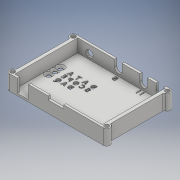
# Autodesk Inventor part: Redid Enclosure Top
Saved by Autodesk Inventor 2017 (Build 210142000, 142)
## iProperties
Created: 2017-07-24
Part Number: Redid Enclosure Top
Material: Generic
Document SubType Name: Modeling
Designer: andrew
Density: 1 g/cm^3
Appearance: Default
Author: andrew
Autodesk Inventor part; units mm, degrees
ref_plane "YZ Plane" through (0, 0, 0) normal (1, 0, 0) x (0, 1, 0)
ref_plane "XZ Plane" through (0, 0, 0) normal (0, 1, 0) x (-1, 0, 0)
ref_plane "XY Plane" through (0, 0, 0) normal (0, 0, 1) x (1, 0, 0)
sketch "Sketch1" plane through (0, 0, 0) normal (0, 0, 1) x (1, 0, 0)
  line L0 (85.72, 30.226) -> (85.72, 1.401) construction
  line L1 (85.72, 1.401) -> (45.72, 1.401) construction
  line L2 (85.72, 1.401) -> (5.72, 1.401) construction
  line L3 (5.72, 1.401) -> (5.72, 59.001) construction
  line L4 (5.72, 59.001) -> (85.72, 59.001) construction
  line L5 (85.72, 59.001) -> (85.72, 1.401) construction
  line L6 (61.99, 1.401) -> (61.99, 20.221) construction
  line L7 (61.99, 20.221) -> (85.72, 20.221) construction
  line L8 (61.99, 20.221) -> (58.44, 20.221) construction
  line L9 (61.99, 23.771) -> (61.99, 20.221) construction
  line L10 (60.215, 20.221) -> (61.99, 20.221) construction
  line L11 (61.99, 20.221) -> (61.99, 21.996) construction
  line L12 (61.99, 21.996) -> (60.215, 21.996) construction
  line L13 (60.215, 21.996) -> (60.215, 20.221) construction
  circle A0 centre (60.215, 21.996) radius 1.775 construction
  circle A1 centre (60.215, 21.996) radius 2.775 construction
  circle A2 centre (60.215, 21.996) radius 4.275 construction
  line L14 (5.72, 59.001) -> (74.72, 59.001) construction
  line L15 (74.72, 59.001) -> (74.72, 53.301) construction
  line L16 (74.72, 53.301) -> (5.72, 53.301) construction
  line L17 (5.72, 53.301) -> (5.72, 59.001) construction
  line L18 (5.72, 1.401) -> (18.72, 1.401) construction
  line L19 (18.72, 1.401) -> (18.72, 14.401) construction
  line L20 (18.72, 14.401) -> (5.72, 14.401) construction
  line L21 (5.72, 14.401) -> (5.72, 1.401) construction
  circle A3 centre (2.72, 58.001) radius 2
  line L22 (3.72, 61.001) -> (5.72, 61.001)
  line L23 (5.72, 61.001) -> (5.72, 59.001) construction
  line L24 (5.72, 61.001) -> (2.72, 61.001)
  line L25 (5.72, 55.001) -> (5.72, 61.001) construction
  line L26 (45.72, 1.9437) -> (45.72, 30.226) construction
  line L27 (45.72, 30.226) -> (85.72, 30.226) construction
  arc A4 (2.72, 61.001) -> (1.52, 55.2515) centre (2.72, 58.001) ccw
  circle A5 centre (2.72, 2.451) radius 2
  line L28 (3.72, -0.549) -> (5.72, -0.549)
  line L29 (5.72, -0.549) -> (2.72, -0.549)
  arc A6 (1.52, 5.2005) -> (2.72, -0.549) centre (2.72, 2.451) ccw
  circle A7 centre (88.72, 58.001) radius 2
  line L30 (85.72, 61.001) -> (88.72, 61.001)
  arc A8 (89.92, 55.2515) -> (88.72, 61.001) centre (88.72, 58.001) ccw
  line L31 (85.72, -0.549) -> (88.72, -0.549)
  circle A9 centre (88.72, 2.451) radius 2
  arc A10 (88.72, -0.549) -> (89.92, 5.2005) centre (88.72, 2.451) ccw
  line L32 (2.72, 53.4184) -> (2.72, 7.0336)
  line L33 (5.72, 61.001) -> (85.72, 61.001)
  line L34 (88.72, 53.4184) -> (88.72, 7.0336)
  line L35 (85.72, -0.549) -> (5.72, -0.549)
  arc A11 (2.72, 53.4184) -> (1.52, 55.2515) centre (0.72, 53.4184) ccw
  arc A12 (1.52, 5.2005) -> (2.72, 7.0336) centre (0.72, 7.0336) ccw
  arc A13 (88.72, 7.0336) -> (89.92, 5.2005) centre (90.72, 7.0336) ccw
  arc A14 (89.92, 55.2515) -> (88.72, 53.4184) centre (90.72, 53.4184) ccw
  point P0 (0, 0)
  point P1 (2.72, 55.001)
  point P2 (2.72, 5.451)
  point P3 (91.44, 0)
  point P4 (88.72, 55.001)
  point P5 (88.72, 5.451)
  dimension "d32" = 40
  dimension "d33" = 28.825
  dimension "d34" = 80
  dimension "d37" = 18.82
  dimension "d40" = 5.55
  dimension "d41" = 8.55
  dimension "d42" = 69
  dimension "d43" = 5.7
  dimension "d44" = 13
  dimension "d45" = 13
  dimension "d52" = 2
  dimension "d80" = 4
  constraints: 72 end point, 20 point on circle, 17 symmetric about line, 14 centre point, 9 parallel, 8 tangent, 7 perpendicular, 6 horizontal, 6 point on line, 3 coincident, 3 equal radius, 2 midpoint, 2 vertical, 1 horizontal alignment, 8 other
  measures "d32" distance of L0.end L1.end
  measures "d33" distance of L0.start L0.end
  measures "d34" distance of L3.end L4.end
  measures "d37" distance of L6.start L6.end
  measures "d40" diameter of A1
  measures "d41" diameter of A2
  measures "d42" distance of L15.end L16.end
  measures "d43" distance of L14.end L15.end
  measures "d44" distance of L20.end L19.end
  measures "d45" distance of L19.end L18.end
  measures "d52" radius of A11
  measures "d80" diameter of A3
extrude "Extrusion1" add sketch "Sketch1" along normal blind 2
sketch "Sketch2" plane through (0, 0, 2) normal (0, 0, 1) x (1, 0, 0)
  line L0 (85.72, 30.226) -> (85.72, 1.401)
  line L1 (5.72, 14.401) -> (5.72, 53.301)
  line L2 (74.72, 59.001) -> (85.72, 59.001)
  line L3 (85.72, 59.001) -> (85.72, 1.401)
  line L4 (45.72, 59.001) -> (74.72, 59.001)
  line L5 (5.72, 58.001) -> (5.72, 59.001)
  line L6 (5.72, 1.401) -> (18.72, 1.401)
  line L7 (5.72, 2.451) -> (5.72, 1.401)
  circle A0 centre (2.72, 58.001) radius 2
  line L8 (3.72, 61.001) -> (5.72, 61.001)
  line L9 (5.72, 61.001) -> (5.72, 59.001)
  line L10 (5.72, 61.001) -> (2.72, 61.001)
  line L11 (5.72, 59.001) -> (5.72, 61.001)
  arc A1 (2.72, 61.001) -> (1.52, 55.2515) centre (2.72, 58.001) ccw
  line L12 (3.72, -0.549) -> (5.72, -0.549)
  line L13 (5.72, -0.549) -> (2.72, -0.549)
  circle A2 centre (2.72, 2.451) radius 2
  arc A3 (1.52, 5.2005) -> (2.72, -0.549) centre (2.72, 2.451) ccw
  line L14 (85.72, -0.549) -> (88.72, -0.549)
  circle A4 centre (88.72, 2.451) radius 2
  arc A5 (88.72, -0.549) -> (89.92, 5.2005) centre (88.72, 2.451) ccw
  circle A6 centre (88.72, 58.001) radius 2
  arc A7 (89.92, 55.2515) -> (88.72, 61.001) centre (88.72, 58.001) ccw
  line L15 (85.72, 61.001) -> (88.72, 61.001)
  line L16 (2.72, 53.4184) -> (2.72, 7.0336)
  line L17 (5.72, 61.001) -> (85.72, 61.001)
  line L18 (88.72, 53.4184) -> (88.72, 7.0336)
  line L19 (85.72, -0.549) -> (5.72, -0.549)
  arc A8 (2.72, 53.4184) -> (1.52, 55.2515) centre (0.72, 53.4184) ccw
  arc A9 (1.52, 5.2005) -> (2.72, 7.0336) centre (0.72, 7.0336) ccw
  arc A10 (88.72, 7.0336) -> (89.92, 5.2005) centre (90.72, 7.0336) ccw
  arc A11 (89.92, 55.2515) -> (88.72, 53.4184) centre (90.72, 53.4184) ccw
  line L20 (85.72, 1.401) -> (74.72, 1.401)
  line L21 (61.99, 1.401) -> (45.72, 1.401)
  line L22 (85.72, 1.401) -> (74.72, 1.401)
  line L23 (61.99, 1.401) -> (18.72, 1.401)
  line L24 (61.99, 1.401) -> (74.72, 1.401)
  line L25 (5.72, 14.401) -> (5.72, 2.451)
  line L26 (5.72, 53.301) -> (5.72, 58.001)
  line L27 (5.72, 59.001) -> (45.72, 59.001)
  point P0 (0, 0)
  point P1 (2.72, 55.001)
  point P2 (2.72, 5.451)
  point P3 (91.44, 0)
  point P4 (88.72, 5.451)
  point P5 (88.72, 55.001)
  dimension "d53" = 40
  dimension "d54" = 28.825
  dimension "d55" = 80
  dimension "d63" = 2
  dimension "d81" = 4
  dimension "d82" = 4
  dimension "d83" = 4
  dimension "d84" = 4
  constraints: 56 end point, 22 point on circle, 12 centre point, 8 tangent, 6 horizontal, 4 parallel, 4 point on line, 3 equal radius, 3 perpendicular, 2 collinear, 2 vertical
  measures "d53" distance of L0.end L21.end
  measures "d54" distance of L0.start L0.end
  measures "d55" distance of L5.end L3.start
  measures "d63" radius of A8
  measures "d81" diameter of A0
  measures "d82" diameter of A2
  measures "d83" diameter of A4
  measures "d84" diameter of A6
extrude "Extrusion2" add sketch "Sketch2" along normal blind 12
sketch "Sketch6" plane through (2.72, 61.001, 0) normal (0, 1, 0) x (1, 0, 0)
  line L0 (36.777, -7.7431) -> (36.777, -7.7246)
  line L1 (43.7769, -7.7246) -> (43.7769, -7.7431)
  arc A0 (43.7769, -7.7431) -> (36.777, -7.7431) centre (40.2769, -7.7227) ccw
  arc A1 (66.82, -7.7246) -> (59.82, -7.7246) centre (63.32, -7.7246) ccw
  arc A2 (81.679, -7.7246) -> (74.679, -7.7246) centre (78.179, -7.7246) ccw
  line L2 (88.72, -8.9422) -> (88.72, 1.0414) construction
  line L3 (-2.72, 0.0414) -> (-2.72, -13.4714) construction
  arc A3 (11.6348, -3.8321) -> (15.9452, -3.8321) centre (13.79, -6.4991) ccw
  line L4 (11.6347, -3.8321) -> (15.9453, -3.8321)
  line L5 (-3, 0) -> (-3, -14) construction
  line L6 (89, 0) -> (89, -14) construction
  line L7 (-3, -7.115) -> (89, -7.115) construction
  line L8 (43, -7.115) -> (43, 6.037) construction
  line L9 (-2.72, -7.115) -> (43, -7.115) construction
  line L10 (47.3567, 23.0307) -> (47.3567, 24.0307)
  line L11 (43, -7.7246) -> (43.7769, -7.7246)
  line L12 (43.7769, -7.7246) -> (43.7769, -19.8521)
  line L13 (43.7769, -19.8521) -> (36.777, -19.8521)
  line L14 (36.777, -19.8521) -> (36.777, -7.7246)
  line L15 (66.82, -7.7246) -> (66.82, -18.3429)
  line L16 (66.82, -18.3429) -> (59.82, -18.3429)
  line L17 (59.82, -18.3429) -> (59.82, -7.7246)
  line L18 (81.679, -7.7246) -> (81.679, -19.1335)
  line L19 (81.679, -19.1335) -> (74.679, -19.1335)
  line L20 (74.679, -19.1335) -> (74.679, -7.7246)
  line L21 (96.4599, -13.1902) -> (96.4599, -14.5902)
  point P0 (-2.72, 0)
  dimension "d91" = 1
  dimension "d92" = 7
  dimension "d93" = 7
  dimension "d94" = 7
  dimension "d141" = 1.4
  constraints: 42 end point, 9 point on circle, 8 point on line, 4 centre point, 4 parallel, 3 vertical, 1 horizontal, 1 midpoint, 1 perpendicular
  measures "d91" distance of L10.start L10.end
  measures "d92" diameter of A0
  measures "d93" diameter of A1
  measures "d94" diameter of A2
  measures "d141" distance of L21.start L21.end
extrude "Extrusion6" cut sketch "Sketch6" against normal blind 10
sketch "Sketch7" plane through (2.72, -0.549, 0) normal (0, -1, 0) x (1, 0, 0)
  line L0 (36.015, 10.636) -> (36.015, 12.9729) construction
  line L1 (7.948, 2) -> (7.948, 12.9729) construction
  line L2 (-2.72, -0.54) -> (-2.72, 13.43) construction
  line L3 (88.72, -0.54) -> (88.72, 12.0462) construction
  line L4 (-2.72, 13.43) -> (88.72, 13.43) construction
  line L5 (43, 13.43) -> (43, 23.4779) construction
  line L6 (0, 14) -> (86, 14) construction
  line L7 (83, 14) -> (3, 14) construction
  line L8 (43, 14) -> (43, 26.0617) construction
  line L9 (36.015, 10.636) -> (36.015, 15.6286)
  line L10 (36.015, 15.6286) -> (49.35, 15.6286)
  line L11 (7.948, 2) -> (7.948, 16.2504)
  line L12 (7.948, 16.2504) -> (17.092, 16.2504)
  line L13 (35.515, 10.8) -> (49.85, 10.8)
  line L14 (49.85, 10.8) -> (49.85, 16.1286)
  line L15 (49.85, 16.1286) -> (35.515, 16.1286)
  line L16 (35.515, 16.1286) -> (35.515, 10.8)
  line L17 (7.448, 2) -> (17.592, 2)
  line L18 (17.592, 2) -> (17.592, 16.7504)
  line L19 (17.592, 16.7504) -> (7.448, 16.7504)
  line L20 (7.448, 16.7504) -> (7.448, 2)
  point P0 (-2.72, 0)
  point P1 (43, 12.16)
  dimension "d101" = 3.2
  dimension "d102" = 12
  constraints: 38 end point, 4 parallel, 2 midpoint, 2 perpendicular, 2 vertical, 1 horizontal, 2 other
  measures "d101" distance between parallel lines of L13 L6
  measures "d102" distance between parallel lines of L6 L17
extrude "Extrusion7" cut sketch "Sketch7" against normal blind 10
sketch "Sketch8" plane through (0, 0, 0) normal (0, 0, -1) x (-1, 0, 0)
  arc A0 (-89.92, 5.2005) -> (-88.72, -0.549) centre (-88.72, 2.451) ccw construction
  line L0 (-91.6567, 1.8381) -> (-82.1567, 1.8381) construction
  line L1 (-20.312, 1.401) -> (-85.72, 1.401) construction
  line L2 (-91.6567, 1.8381) -> (-82.1567, 1.8381) construction
  line L3 (-82.1567, -0.549) -> (-82.1567, 5.751) construction
  line L4 (-82.1567, 5.751) -> (-78.6567, 5.751) construction
  line L5 (-78.6567, 5.751) -> (-78.6567, 9.251) construction
  line L6 (-78.6567, 9.251) -> (-82.1567, 9.251) construction
  line L7 (-82.1567, 9.251) -> (-82.1567, 5.751) construction
  circle A1 centre (-80.4067, 7.501) radius 1.75
  line L8 (-84.399, 59.001) -> (-77.399, 59.001) construction
  line L9 (-84.399, 61.001) -> (-84.399, 59.001) construction
  line L10 (-77.399, 61.001) -> (-84.399, 61.001) construction
  line L11 (-77.399, 61.001) -> (-77.399, 59.001) construction
  line L12 (-69.54, 59.001) -> (-62.54, 59.001) construction
  line L13 (-69.54, 61.001) -> (-69.54, 59.001) construction
  line L14 (-62.54, 61.001) -> (-69.54, 61.001) construction
  line L15 (-62.54, 61.001) -> (-62.54, 59.001) construction
  line L16 (-46.4969, 59.001) -> (-39.497, 59.001) construction
  line L17 (-46.4969, 61.001) -> (-46.4969, 59.001) construction
  line L18 (-39.497, 61.001) -> (-46.4969, 61.001) construction
  line L19 (-39.497, 61.001) -> (-39.497, 59.001) construction
  line L20 (-88.72, 61.001) -> (-2.72, 61.001) construction
  line L21 (-80.899, 61.001) -> (-80.899, 58.001) construction
  line L22 (-80.899, 61.001) -> (-77.899, 61.001) construction
  line L23 (-66.04, 61.001) -> (-66.04, 58.001) construction
  line L24 (-42.9969, 61.001) -> (-42.9969, 58.001) construction
  line L25 (-81.6541, 57.9429) -> (-78.5881, 57.9429) construction
  line L26 (-78.5881, 57.9429) -> (-78.5881, 54.4344) construction
  line L27 (-78.5881, 54.4344) -> (-81.6541, 54.4344) construction
  line L28 (-81.6541, 54.4344) -> (-81.6541, 57.9429) construction
  line L29 (-44.9835, 57.8582) -> (-36.2955, 57.8582) construction
  line L30 (-36.2955, 57.8582) -> (-36.2955, 54.005) construction
  line L31 (-36.2955, 54.005) -> (-44.9835, 54.005) construction
  line L32 (-44.9835, 54.005) -> (-44.9835, 57.8582) construction
  line L33 (-68.3878, 54.2701) -> (-68.3878, 58.1234) construction
  line L34 (-68.3878, 58.1234) -> (-59.6998, 58.1234) construction
  line L35 (-59.6998, 58.1234) -> (-59.6998, 54.2701) construction
  line L36 (-59.6998, 54.2701) -> (-68.3878, 54.2701) construction
  arc A2 (-1.52, 55.2515) -> (-2.72, 61.001) centre (-2.72, 58.001) ccw construction
  line L37 (0.28, 58.001) -> (-7.5071, 58.001) construction
  line L38 (-85.72, 59.001) -> (-5.72, 59.001) construction
  line L39 (0.28, 58.001) -> (8.0671, 58.001) construction
  line L40 (-7.5071, 61.001) -> (-7.5071, 41.501) construction
  line L41 (-7.5071, 41.501) -> (-11.0671, 41.501) construction
  line L42 (-11.0671, 41.501) -> (-11.0671, 37.941) construction
  line L43 (-11.0671, 37.941) -> (-7.5071, 37.941) construction
  line L44 (-7.5071, 37.941) -> (-7.5071, 41.501) construction
  line L45 (-7.5071, 61.001) -> (-7.5071, 36.381) construction
  line L46 (-7.5071, 61.001) -> (17.1129, 61.001) construction
  line L47 (-7.5071, 36.381) -> (-11.0671, 36.381) construction
  line L48 (-11.0671, 36.381) -> (-11.0671, 32.821) construction
  line L49 (-11.0671, 32.821) -> (-7.5071, 32.821) construction
  line L50 (-7.5071, 32.821) -> (-7.5071, 36.381) construction
  line L51 (-7.5071, 61.001) -> (-7.5071, 30.621) construction
  line L52 (-7.5071, 30.621) -> (-11.0671, 30.621) construction
  line L53 (-11.0671, 30.621) -> (-11.0671, 27.061) construction
  line L54 (-11.0671, 27.061) -> (-7.5071, 27.061) construction
  line L55 (-7.5071, 27.061) -> (-7.5071, 30.621) construction
  circle A3 centre (-9.2871, 39.721) radius 1.78
  circle A4 centre (-9.2871, 34.601) radius 1.78
  circle A5 centre (-9.2871, 28.841) radius 1.78
  line L56 (-42.0074, 37.4126) -> (-42.0074, 41.2658) construction
  line L57 (-42.0074, 41.2658) -> (-11.5337, 41.2658) construction
  line L58 (-11.5337, 41.2658) -> (-11.5337, 37.4126) construction
  line L59 (-11.5337, 37.4126) -> (-42.0074, 37.4126) construction
  line L60 (-41.4894, 32.436) -> (-41.4894, 36.2892) construction
  line L61 (-41.4894, 36.2892) -> (-11.0157, 36.2892) construction
  line L62 (-11.0157, 36.2892) -> (-11.0157, 32.436) construction
  line L63 (-11.0157, 32.436) -> (-41.4894, 32.436) construction
  line L64 (-31.8137, 26.6882) -> (-31.8137, 30.5415) construction
  line L65 (-31.8137, 30.5415) -> (-1.34, 30.5415) construction
  line L66 (-1.34, 30.5415) -> (-1.34, 26.6882) construction
  line L67 (-1.34, 26.6882) -> (-31.8137, 26.6882) construction
  line L68 (-80.3543, 53.7647) -> (-81.2943, 53.7647)
  line L69 (-81.2943, 53.7647) -> (-81.2943, 57.9429)
  line L70 (-81.2943, 57.9429) -> (-80.3543, 57.9429)
  line L71 (-80.3543, 57.9429) -> (-80.3543, 53.7647)
  line L72 (-67.088, 53.9451) -> (-68.028, 53.9451)
  line L73 (-68.028, 53.9451) -> (-68.028, 58.1234)
  line L74 (-68.028, 58.1234) -> (-67.088, 58.1234)
  line L75 (-67.088, 58.1234) -> (-67.088, 53.9451)
  line L76 (-63.8173, 53.9451) -> (-64.7574, 53.9451)
  line L77 (-64.7574, 53.9451) -> (-64.7574, 58.1234)
  line L78 (-64.7574, 58.1234) -> (-63.8173, 58.1234)
  line L79 (-63.8173, 58.1234) -> (-63.8173, 53.9451)
  spline S0 degree 2 poles (-43.3336, 53.7156) (-43.7939, 53.7156) (-44.4876, 53.8939) (-44.7858, 54.0235) knots 0 0 0 1 2 2 2
  line L80 (-44.7858, 54.0235) -> (-44.7858, 54.9765)
  line L81 (-44.7858, 54.9765) -> (-44.695, 54.9765)
  spline S1 degree 2 poles (-44.695, 54.9765) (-44.3936, 54.7205) (-43.6707, 54.4449) (-43.3304, 54.4449) knots 0 0 0 1 2 2 2
  spline S2 degree 2 poles (-43.3304, 54.4449) (-43.2428, 54.4449) (-42.9608, 54.4838) (-42.8765, 54.5227) knots 0 0 0 1 2 2 2
  spline S3 degree 2 poles (-42.8765, 54.5227) (-42.7728, 54.5681) (-42.627, 54.7334) (-42.627, 54.8663) knots 0 0 0 1 2 2 2
  spline S4 degree 2 poles (-42.627, 54.8663) (-42.627, 55.0187) (-42.8636, 55.2067) (-43.0257, 55.2488) knots 0 0 0 1 2 2 2
  spline S5 degree 2 poles (-43.0257, 55.2488) (-43.2299, 55.3039) (-43.6934, 55.3979) (-43.8976, 55.4693) knots 0 0 0 1 2 2 2
  spline S6 degree 2 poles (-43.8976, 55.4693) (-44.3612, 55.6313) (-44.7631, 56.1856) (-44.7631, 56.6005) knots 0 0 0 1 2 2 2
  spline S7 degree 2 poles (-44.7631, 56.6005) (-44.7631, 57.1613) (-43.8133, 57.8582) (-43.1002, 57.8582) knots 0 0 0 1 2 2 2
  spline S8 degree 2 poles (-43.1002, 57.8582) (-42.7436, 57.8582) (-42.037, 57.7124) (-41.7582, 57.5892) knots 0 0 0 1 2 2 2
  line L82 (-41.7582, 57.5892) -> (-41.7582, 56.6751)
  line L83 (-41.7582, 56.6751) -> (-41.8458, 56.6751)
  spline S9 degree 2 poles (-41.8458, 56.6751) (-42.0694, 56.8663) (-42.7112, 57.1289) (-43.0483, 57.1289) knots 0 0 0 1 2 2 2
  spline S10 degree 2 poles (-43.0483, 57.1289) (-43.1812, 57.1289) (-43.3887, 57.09) (-43.5054, 57.0381) knots 0 0 0 1 2 2 2
  spline S11 degree 2 poles (-43.5054, 57.0381) (-43.5994, 56.996) (-43.7355, 56.8274) (-43.7355, 56.7237) knots 0 0 0 1 2 2 2
  spline S12 degree 2 poles (-43.7355, 56.7237) (-43.7355, 56.5681) (-43.5184, 56.3898) (-43.2072, 56.3185) knots 0 0 0 1 2 2 2
  spline S13 degree 2 poles (-43.2072, 56.3185) (-43.0062, 56.2731) (-42.6334, 56.1856) (-42.4195, 56.1111) knots 0 0 0 1 2 2 2
  spline S14 degree 2 poles (-42.4195, 56.1111) (-42.0046, 55.9587) (-41.5994, 55.453) (-41.5994, 55.0381) knots 0 0 0 1 2 2 2
  spline S15 degree 2 poles (-41.5994, 55.0381) (-41.5994, 54.4417) (-42.5362, 53.7156) (-43.3336, 53.7156) knots 0 0 0 1 2 2 2
  spline S16 degree 2 poles (-38.0236, 39.2626) (-38.0236, 38.7018) (-38.5131, 37.8201) (-38.8858, 37.5835) knots 0 0 0 1 2 2 2
  spline S17 degree 2 poles (-38.8858, 37.5835) (-39.197, 37.3825) (-39.9296, 37.2658) (-40.3413, 37.2658) knots 0 0 0 1 2 2 2
  line L84 (-40.3413, 37.2658) -> (-41.5925, 37.2658)
  line L85 (-41.5925, 37.2658) -> (-41.5925, 41.2658)
  line L86 (-41.5925, 41.2658) -> (-40.3542, 41.2658)
  spline S18 degree 2 poles (-40.3542, 41.2658) (-39.9328, 41.2658) (-39.197, 41.1589) (-38.8729, 40.9514) knots 0 0 0 1 2 2 2
  spline S19 degree 2 poles (-38.8729, 40.9514) (-38.4806, 40.6986) (-38.0236, 39.8428) (-38.0236, 39.2626) knots 0 0 0 1 2 2 2
  spline S20 degree 2 poles (-39.0544, 39.2691) (-39.0544, 39.6645) (-39.3267, 40.2286) (-39.6054, 40.3874) knots 0 0 0 1 2 2 2
  spline S21 degree 2 poles (-39.6054, 40.3874) (-39.8097, 40.4976) (-40.257, 40.5203) (-40.5682, 40.5203) knots 0 0 0 1 2 2 2
  line L87 (-40.5682, 40.5203) -> (-40.5876, 40.5203)
  line L88 (-40.5876, 40.5203) -> (-40.5876, 38.0146)
  line L89 (-40.5876, 38.0146) -> (-40.5682, 38.0146)
  spline S22 degree 2 poles (-40.5682, 38.0146) (-40.231, 38.0146) (-39.7675, 38.0373) (-39.5568, 38.1702) knots 0 0 0 1 2 2 2
  spline S23 degree 2 poles (-39.5568, 38.1702) (-39.3105, 38.3258) (-39.0544, 38.8736) (-39.0544, 39.2691) knots 0 0 0 1 2 2 2
  line L90 (-34.6362, 37.2658) -> (-33.2845, 41.2658)
  line L91 (-33.2845, 41.2658) -> (-32.1889, 41.2658)
  line L92 (-32.1889, 41.2658) -> (-30.8372, 37.2658)
  line L93 (-30.8372, 37.2658) -> (-31.8712, 37.2658)
  line L94 (-31.8712, 37.2658) -> (-32.1208, 38.0827)
  line L95 (-32.1208, 38.0827) -> (-33.3785, 38.0827)
  line L96 (-33.3785, 38.0827) -> (-33.6314, 37.2658)
  line L97 (-33.6314, 37.2658) -> (-34.6362, 37.2658)
  line L98 (-32.3413, 38.8088) -> (-32.7497, 40.1313)
  line L99 (-32.7497, 40.1313) -> (-33.1614, 38.8088)
  line L100 (-33.1614, 38.8088) -> (-32.3413, 38.8088)
  line L101 (-26.4482, 37.2658) -> (-26.4482, 40.5041)
  line L102 (-26.4482, 40.5041) -> (-27.6314, 40.5041)
  line L103 (-27.6314, 40.5041) -> (-27.6314, 41.2658)
  line L104 (-27.6314, 41.2658) -> (-24.2602, 41.2658)
  line L105 (-24.2602, 41.2658) -> (-24.2602, 40.5041)
  line L106 (-24.2602, 40.5041) -> (-25.4434, 40.5041)
  line L107 (-25.4434, 40.5041) -> (-25.4434, 37.2658)
  line L108 (-25.4434, 37.2658) -> (-26.4482, 37.2658)
  line L109 (-21.0576, 37.2658) -> (-19.7059, 41.2658)
  line L110 (-19.7059, 41.2658) -> (-18.6103, 41.2658)
  line L111 (-18.6103, 41.2658) -> (-17.2586, 37.2658)
  line L112 (-17.2586, 37.2658) -> (-18.2926, 37.2658)
  line L113 (-18.2926, 37.2658) -> (-18.5422, 38.0827)
  line L114 (-18.5422, 38.0827) -> (-19.7999, 38.0827)
  line L115 (-19.7999, 38.0827) -> (-20.0528, 37.2658)
  line L116 (-20.0528, 37.2658) -> (-21.0576, 37.2658)
  line L117 (-18.7627, 38.8088) -> (-19.1711, 40.1313)
  line L118 (-19.1711, 40.1313) -> (-19.5828, 38.8088)
  line L119 (-19.5828, 38.8088) -> (-18.7627, 38.8088)
  spline S24 degree 2 poles (-39.8395, 32.1337) (-40.2997, 32.1337) (-40.9934, 32.3119) (-41.2916, 32.4416) knots 0 0 0 1 2 2 2
  line L120 (-41.2916, 32.4416) -> (-41.2916, 33.3946)
  line L121 (-41.2916, 33.3946) -> (-41.2009, 33.3946)
  spline S25 degree 2 poles (-41.2009, 33.3946) (-40.8994, 33.1385) (-40.1766, 32.863) (-39.8362, 32.863) knots 0 0 0 1 2 2 2
  spline S26 degree 2 poles (-39.8362, 32.863) (-39.7487, 32.863) (-39.4667, 32.9019) (-39.3824, 32.9408) knots 0 0 0 1 2 2 2
  spline S27 degree 2 poles (-39.3824, 32.9408) (-39.2787, 32.9862) (-39.1328, 33.1515) (-39.1328, 33.2844) knots 0 0 0 1 2 2 2
  spline S28 degree 2 poles (-39.1328, 33.2844) (-39.1328, 33.4367) (-39.3694, 33.6247) (-39.5315, 33.6669) knots 0 0 0 1 2 2 2
  spline S29 degree 2 poles (-39.5315, 33.6669) (-39.7357, 33.722) (-40.1993, 33.816) (-40.4035, 33.8873) knots 0 0 0 1 2 2 2
  spline S30 degree 2 poles (-40.4035, 33.8873) (-40.867, 34.0494) (-41.2689, 34.6037) (-41.2689, 35.0186) knots 0 0 0 1 2 2 2
  spline S31 degree 2 poles (-41.2689, 35.0186) (-41.2689, 35.5794) (-40.3192, 36.2763) (-39.6061, 36.2763) knots 0 0 0 1 2 2 2
  spline S32 degree 2 poles (-39.6061, 36.2763) (-39.2495, 36.2763) (-38.5429, 36.1304) (-38.2641, 36.0072) knots 0 0 0 1 2 2 2
  line L122 (-38.2641, 36.0072) -> (-38.2641, 35.0931)
  line L123 (-38.2641, 35.0931) -> (-38.3516, 35.0931)
  spline S33 degree 2 poles (-38.3516, 35.0931) (-38.5753, 35.2844) (-39.2171, 35.5469) (-39.5542, 35.5469) knots 0 0 0 1 2 2 2
  spline S34 degree 2 poles (-39.5542, 35.5469) (-39.6871, 35.5469) (-39.8946, 35.508) (-40.0112, 35.4562) knots 0 0 0 1 2 2 2
  spline S35 degree 2 poles (-40.0112, 35.4562) (-40.1053, 35.414) (-40.2414, 35.2455) (-40.2414, 35.1418) knots 0 0 0 1 2 2 2
  spline S36 degree 2 poles (-40.2414, 35.1418) (-40.2414, 34.9862) (-40.0242, 34.8079) (-39.713, 34.7366) knots 0 0 0 1 2 2 2
  spline S37 degree 2 poles (-39.713, 34.7366) (-39.5121, 34.6912) (-39.1393, 34.6037) (-38.9253, 34.5291) knots 0 0 0 1 2 2 2
  spline S38 degree 2 poles (-38.9253, 34.5291) (-38.5104, 34.3768) (-38.1053, 33.8711) (-38.1053, 33.4562) knots 0 0 0 1 2 2 2
  spline S39 degree 2 poles (-38.1053, 33.4562) (-38.1053, 32.8598) (-39.042, 32.1337) (-39.8395, 32.1337) knots 0 0 0 1 2 2 2
  spline S40 degree 2 poles (-34.2544, 32.1272) (-35.1555, 32.1272) (-36.2122, 33.2163) (-36.2122, 34.2017) knots 0 0 0 1 2 2 2
  spline S41 degree 2 poles (-36.2122, 34.2017) (-36.2122, 35.1515) (-35.1523, 36.2828) (-34.2511, 36.2828) knots 0 0 0 1 2 2 2
  spline S42 degree 2 poles (-34.2511, 36.2828) (-34.0145, 36.2828) (-33.632, 36.2277) (-33.457, 36.1823) knots 0 0 0 1 2 2 2
  spline S43 degree 2 poles (-33.457, 36.1823) (-33.3208, 36.1401) (-32.9999, 36.0008) (-32.8994, 35.9489) knots 0 0 0 1 2 2 2
  line L124 (-32.8994, 35.9489) -> (-32.8994, 34.9959)
  line L125 (-32.8994, 34.9959) -> (-32.9999, 34.9959)
  spline S44 degree 2 poles (-32.9999, 34.9959) (-33.0745, 35.0607) (-33.2949, 35.2422) (-33.4343, 35.3265) knots 0 0 0 1 2 2 2
  spline S45 degree 2 poles (-33.4343, 35.3265) (-33.5736, 35.414) (-33.9075, 35.534) (-34.0923, 35.534) knots 0 0 0 1 2 2 2
  spline S46 degree 2 poles (-34.0923, 35.534) (-34.3095, 35.534) (-34.6693, 35.3978) (-34.8346, 35.226) knots 0 0 0 1 2 2 2
  spline S47 degree 2 poles (-34.8346, 35.226) (-34.9837, 35.0737) (-35.1749, 34.5518) (-35.1749, 34.1985) knots 0 0 0 1 2 2 2
  spline S48 degree 2 poles (-35.1749, 34.1985) (-35.1749, 33.8257) (-34.9772, 33.3168) (-34.8151, 33.1612) knots 0 0 0 1 2 2 2
  spline S49 degree 2 poles (-34.8151, 33.1612) (-34.6595, 33.0089) (-34.2771, 32.876) (-34.0858, 32.876) knots 0 0 0 1 2 2 2
  spline S50 degree 2 poles (-34.0858, 32.876) (-33.8881, 32.876) (-33.5283, 33.0089) (-33.4051, 33.0899) knots 0 0 0 1 2 2 2
  spline S51 degree 2 poles (-33.4051, 33.0899) (-33.2689, 33.1709) (-33.0647, 33.3427) (-32.9902, 33.4108) knots 0 0 0 1 2 2 2
  line L126 (-32.9902, 33.4108) -> (-32.8994, 33.4108)
  line L127 (-32.8994, 33.4108) -> (-32.8994, 32.4708)
  spline S52 degree 2 poles (-32.8994, 32.4708) (-33.0096, 32.4189) (-33.2981, 32.2892) (-33.4537, 32.2439) knots 0 0 0 1 2 2 2
  spline S53 degree 2 poles (-33.4537, 32.2439) (-33.6417, 32.1855) (-33.9691, 32.1272) (-34.2544, 32.1272) knots 0 0 0 1 2 2 2
  spline S54 degree 2 poles (-27.055, 34.205) (-27.055, 33.2325) (-28.0923, 32.1207) (-28.9934, 32.1207) knots 0 0 0 1 2 2 2
  spline S55 degree 2 poles (-28.9934, 32.1207) (-29.8978, 32.1207) (-30.9286, 33.2455) (-30.9286, 34.205) knots 0 0 0 1 2 2 2
  spline S56 degree 2 poles (-30.9286, 34.205) (-30.9286, 35.1677) (-29.8978, 36.2892) (-28.9934, 36.2892) knots 0 0 0 1 2 2 2
  spline S57 degree 2 poles (-28.9934, 36.2892) (-28.0923, 36.2892) (-27.055, 35.1742) (-27.055, 34.205) knots 0 0 0 1 2 2 2
  spline S58 degree 2 poles (-28.0923, 34.205) (-28.0923, 34.5648) (-28.2382, 35.0672) (-28.3646, 35.226) knots 0 0 0 1 2 2 2
  spline S59 degree 2 poles (-28.3646, 35.226) (-28.491, 35.3914) (-28.8151, 35.534) (-28.9902, 35.534) knots 0 0 0 1 2 2 2
  spline S60 degree 2 poles (-28.9902, 35.534) (-29.1749, 35.534) (-29.4764, 35.4011) (-29.6158, 35.2325) knots 0 0 0 1 2 2 2
  spline S61 degree 2 poles (-29.6158, 35.2325) (-29.739, 35.0769) (-29.8913, 34.5615) (-29.8913, 34.205) knots 0 0 0 1 2 2 2
  spline S62 degree 2 poles (-29.8913, 34.205) (-29.8913, 33.8354) (-29.7454, 33.3492) (-29.619, 33.1839) knots 0 0 0 1 2 2 2
  spline S63 degree 2 poles (-29.619, 33.1839) (-29.4926, 33.0186) (-29.1652, 32.876) (-28.9902, 32.876) knots 0 0 0 1 2 2 2
  spline S64 degree 2 poles (-28.9902, 32.876) (-28.8119, 32.876) (-28.4813, 33.0283) (-28.3613, 33.1904) knots 0 0 0 1 2 2 2
  spline S65 degree 2 poles (-28.3613, 33.1904) (-28.2317, 33.3654) (-28.0923, 33.829) (-28.0923, 34.205) knots 0 0 0 1 2 2 2
  spline S66 degree 2 poles (-21.7714, 34.944) (-21.7714, 34.6653) (-21.9497, 34.1596) (-22.115, 33.991) knots 0 0 0 1 2 2 2
  spline S67 degree 2 poles (-22.115, 33.991) (-22.2155, 33.8841) (-22.4618, 33.709) (-22.6077, 33.6474) knots 0 0 0 1 2 2 2
  spline S68 degree 2 poles (-22.6077, 33.6474) (-22.7568, 33.5858) (-23.1036, 33.5145) (-23.3176, 33.5145) knots 0 0 0 1 2 2 2
  line L128 (-23.3176, 33.5145) -> (-23.8427, 33.5145)
  line L129 (-23.8427, 33.5145) -> (-23.8427, 32.205)
  line L130 (-23.8427, 32.205) -> (-24.8476, 32.205)
  line L131 (-24.8476, 32.205) -> (-24.8476, 36.205)
  line L132 (-24.8476, 36.205) -> (-23.2949, 36.205)
  spline S69 degree 2 poles (-23.2949, 36.205) (-22.9513, 36.205) (-22.4489, 36.0786) (-22.2446, 35.9424) knots 0 0 0 1 2 2 2
  spline S70 degree 2 poles (-22.2446, 35.9424) (-22.0177, 35.7901) (-21.7714, 35.2909) (-21.7714, 34.944) knots 0 0 0 1 2 2 2
  spline S71 degree 2 poles (-22.8022, 34.9181) (-22.8022, 35.0899) (-22.9642, 35.333) (-23.0745, 35.3784) knots 0 0 0 1 2 2 2
  spline S72 degree 2 poles (-23.0745, 35.3784) (-23.2171, 35.44) (-23.4764, 35.4594) (-23.7001, 35.4594) knots 0 0 0 1 2 2 2
  line L133 (-23.7001, 35.4594) -> (-23.8427, 35.4594)
  line L134 (-23.8427, 35.4594) -> (-23.8427, 34.2601)
  line L135 (-23.8427, 34.2601) -> (-23.7714, 34.2601)
  spline S73 degree 2 poles (-23.7714, 34.2601) (-23.632, 34.2601) (-23.3792, 34.2666) (-23.2852, 34.2828) knots 0 0 0 1 2 2 2
  spline S74 degree 2 poles (-23.2852, 34.2828) (-23.2041, 34.2957) (-23.0258, 34.3735) (-22.9772, 34.4222) knots 0 0 0 1 2 2 2
  spline S75 degree 2 poles (-22.9772, 34.4222) (-22.8735, 34.5194) (-22.8022, 34.7366) (-22.8022, 34.9181) knots 0 0 0 1 2 2 2
  line L136 (-19.6223, 32.205) -> (-19.6223, 36.205)
  line L137 (-19.6223, 36.205) -> (-16.9189, 36.205)
  line L138 (-16.9189, 36.205) -> (-16.9189, 35.4432)
  line L139 (-16.9189, 35.4432) -> (-18.6239, 35.4432)
  line L140 (-18.6239, 35.4432) -> (-18.6239, 34.7398)
  line L141 (-18.6239, 34.7398) -> (-17.0518, 34.7398)
  line L142 (-17.0518, 34.7398) -> (-17.0518, 33.9781)
  line L143 (-17.0518, 33.9781) -> (-18.6239, 33.9781)
  line L144 (-18.6239, 33.9781) -> (-18.6239, 32.9667)
  line L145 (-18.6239, 32.9667) -> (-16.9189, 32.9667)
  line L146 (-16.9189, 32.9667) -> (-16.9189, 32.205)
  line L147 (-16.9189, 32.205) -> (-19.6223, 32.205)
  spline S76 degree 2 poles (-27.8299, 28.454) (-27.8299, 27.8932) (-28.3193, 27.0115) (-28.6921, 26.7749) knots 0 0 0 1 2 2 2
  spline S77 degree 2 poles (-28.6921, 26.7749) (-29.0033, 26.5739) (-29.7359, 26.4572) (-30.1475, 26.4572) knots 0 0 0 1 2 2 2
  line L148 (-30.1475, 26.4572) -> (-31.3988, 26.4572)
  line L149 (-31.3988, 26.4572) -> (-31.3988, 30.4572)
  line L150 (-31.3988, 30.4572) -> (-30.1605, 30.4572)
  spline S78 degree 2 poles (-30.1605, 30.4572) (-29.7391, 30.4572) (-29.0033, 30.3502) (-28.6791, 30.1428) knots 0 0 0 1 2 2 2
  spline S79 degree 2 poles (-28.6791, 30.1428) (-28.2869, 29.8899) (-27.8299, 29.0342) (-27.8299, 28.454) knots 0 0 0 1 2 2 2
  spline S80 degree 2 poles (-28.8607, 28.4604) (-28.8607, 28.8559) (-29.133, 29.4199) (-29.4117, 29.5788) knots 0 0 0 1 2 2 2
  spline S81 degree 2 poles (-29.4117, 29.5788) (-29.6159, 29.689) (-30.0633, 29.7117) (-30.3744, 29.7117) knots 0 0 0 1 2 2 2
  line L151 (-30.3744, 29.7117) -> (-30.3939, 29.7117)
  line L152 (-30.3939, 29.7117) -> (-30.3939, 27.206)
  line L153 (-30.3939, 27.206) -> (-30.3744, 27.206)
  spline S82 degree 2 poles (-30.3744, 27.206) (-30.0373, 27.206) (-29.5738, 27.2287) (-29.3631, 27.3616) knots 0 0 0 1 2 2 2
  spline S83 degree 2 poles (-29.3631, 27.3616) (-29.1168, 27.5172) (-28.8607, 28.065) (-28.8607, 28.4604) knots 0 0 0 1 2 2 2
  line L154 (-26.0535, 26.4572) -> (-24.7018, 30.4572)
  line L155 (-24.7018, 30.4572) -> (-23.6062, 30.4572)
  line L156 (-23.6062, 30.4572) -> (-22.2545, 26.4572)
  line L157 (-22.2545, 26.4572) -> (-23.2885, 26.4572)
  line L158 (-23.2885, 26.4572) -> (-23.5381, 27.2741)
  line L159 (-23.5381, 27.2741) -> (-24.7958, 27.2741)
  line L160 (-24.7958, 27.2741) -> (-25.0487, 26.4572)
  line L161 (-25.0487, 26.4572) -> (-26.0535, 26.4572)
  line L162 (-23.7586, 28.0002) -> (-24.167, 29.3227)
  line L163 (-24.167, 29.3227) -> (-24.5787, 28.0002)
  line L164 (-24.5787, 28.0002) -> (-23.7586, 28.0002)
  spline S84 degree 2 poles (-16.6111, 25.4005) (-16.7732, 25.3616) (-17.0973, 25.3227) (-17.4441, 25.3227) knots 0 0 0 1 2 2 2
  spline S85 degree 2 poles (-17.4441, 25.3227) (-17.7586, 25.3227) (-18.2026, 25.4815) (-18.3518, 25.6274) knots 0 0 0 1 2 2 2
  spline S86 degree 2 poles (-18.3518, 25.6274) (-18.4976, 25.77) (-18.6467, 26.159) (-18.6565, 26.3859) knots 0 0 0 1 2 2 2
  spline S87 degree 2 poles (-18.6565, 26.3859) (-19.5025, 26.4248) (-20.4782, 27.5237) (-20.4782, 28.4572) knots 0 0 0 1 2 2 2
  spline S88 degree 2 poles (-20.4782, 28.4572) (-20.4782, 29.4199) (-19.4474, 30.5415) (-18.543, 30.5415) knots 0 0 0 1 2 2 2
  spline S89 degree 2 poles (-18.543, 30.5415) (-17.6419, 30.5415) (-16.6046, 29.4264) (-16.6046, 28.4572) knots 0 0 0 1 2 2 2
  spline S90 degree 2 poles (-16.6046, 28.4572) (-16.6046, 27.7506) (-17.1913, 26.7392) (-17.7294, 26.5253) knots 0 0 0 1 2 2 2
  spline S91 degree 2 poles (-17.7294, 26.5253) (-17.7229, 26.2303) (-17.4733, 26.0066) (-17.1621, 26.0066) knots 0 0 0 1 2 2 2
  spline S92 degree 2 poles (-17.1621, 26.0066) (-17.039, 26.0066) (-16.7699, 26.078) (-16.7116, 26.1104) knots 0 0 0 1 2 2 2
  line L165 (-16.7116, 26.1104) -> (-16.6111, 26.1104)
  line L166 (-16.6111, 26.1104) -> (-16.6111, 25.4005)
  spline S93 degree 2 poles (-17.9109, 27.4459) (-17.7813, 27.6209) (-17.6419, 28.0844) (-17.6419, 28.4604) knots 0 0 0 1 2 2 2
  spline S94 degree 2 poles (-17.6419, 28.4604) (-17.6419, 28.817) (-17.7877, 29.3194) (-17.9142, 29.4815) knots 0 0 0 1 2 2 2
  spline S95 degree 2 poles (-17.9142, 29.4815) (-18.0406, 29.6436) (-18.3647, 29.7862) (-18.5398, 29.7862) knots 0 0 0 1 2 2 2
  spline S96 degree 2 poles (-18.5398, 29.7862) (-18.7245, 29.7862) (-19.026, 29.6533) (-19.1654, 29.4848) knots 0 0 0 1 2 2 2
  spline S97 degree 2 poles (-19.1654, 29.4848) (-19.2885, 29.3292) (-19.4409, 28.8138) (-19.4409, 28.4572) knots 0 0 0 1 2 2 2
  spline S98 degree 2 poles (-19.4409, 28.4572) (-19.4409, 28.0909) (-19.295, 27.6047) (-19.1686, 27.4394) knots 0 0 0 1 2 2 2
  spline S99 degree 2 poles (-19.1686, 27.4394) (-19.0422, 27.2741) (-18.7148, 27.1314) (-18.5398, 27.1314) knots 0 0 0 1 2 2 2
  spline S100 degree 2 poles (-18.5398, 27.1314) (-18.3615, 27.1314) (-18.0309, 27.2838) (-17.9109, 27.4459) knots 0 0 0 1 2 2 2
  point P0 (0, 0)
  dimension "d103" = 9.5
  dimension "d104" = 0
  dimension "d105" = 6.3
  dimension "d106" = 3.5
  dimension "d107" = 3.5
  dimension "d108" = 3
  dimension "d109" = 90
  dimension "d110" = 7.7871
  dimension "d111" = 180
  dimension "d112" = 19.5
  dimension "d113" = 3.56
  dimension "d114" = 3.56
  dimension "d115" = 24.62
  dimension "d116" = 90
  dimension "d117" = 3.56
  dimension "d118" = 3.56
  dimension "d119" = 30.38
  dimension "d120" = 3.56
  dimension "d121" = 3.56
  constraints: 58 end point, 10 parallel, 8 horizontal, 6 vertical, 5 perpendicular, 4 centre point, 4 equal length, 2 point on circle, 2 tangent, 17 other
  measures "d103" distance of L0.start L0.end
  measures "d104" distance between parallel lines of L0 L2
  measures "d105" distance of L3.start L3.end
  measures "d106" distance of L6.end L5.end
  measures "d107" distance of L5.end L4.end
  measures "d108" distance of L21.start L21.end
  measures "d109" angle of L21 L22
  measures "d110" distance of L37.start L37.end
  measures "d111" angle of L37 L39
  measures "d112" distance of L40.start L40.end
  measures "d113" distance of L43.end L42.end
  measures "d114" distance of L42.end L41.end
  measures "d115" distance of L40.start L45.end
  measures "d116" angle of L45 L46
  measures "d117" distance of L49.end L48.end
  measures "d118" distance of L48.end L47.end
  measures "d119" distance of L40.start L51.end
  measures "d120" distance of L54.end L53.end
  measures "d121" distance of L53.end L52.end
extrude "Extrusion8" cut sketch "Sketch8" against normal blind 10
sketch "Sketch9" plane through (0, 0, 0) normal (0, 0, -1) x (-1, 0, 0)
  spline S0 degree 2 poles (-39.6054, 40.3874) (-39.8097, 40.4976) (-40.257, 40.5203) (-40.5682, 40.5203) knots 0 0 0 0.5 1 1 1 projected
  line L0 (-40.5682, 40.5203) -> (-40.5876, 40.5203) projected
  line L1 (-40.5876, 40.5203) -> (-40.5876, 38.0146) projected
  line L2 (-40.5876, 38.0146) -> (-40.5682, 38.0146) projected
  spline S1 degree 2 poles (-40.5682, 38.0146) (-40.231, 38.0146) (-39.7675, 38.0373) (-39.5568, 38.1702) knots 0 0 0 0.5 1 1 1 projected
  spline S2 degree 2 poles (-39.5568, 38.1702) (-39.3105, 38.3258) (-39.0544, 38.8736) (-39.0544, 39.2691) knots 0 0 0 0.5 1 1 1 projected
  spline S3 degree 2 poles (-39.0544, 39.2691) (-39.0544, 39.6645) (-39.3267, 40.2286) (-39.6054, 40.3874) knots 0 0 0 0.5 1 1 1 projected
  line L3 (-32.7497, 40.1313) -> (-33.1614, 38.8088) projected
  line L4 (-33.1614, 38.8088) -> (-32.3413, 38.8088) projected
  line L5 (-32.3413, 38.8088) -> (-32.7497, 40.1313) projected
  line L6 (-19.1711, 40.1313) -> (-19.5828, 38.8088) projected
  line L7 (-19.5828, 38.8088) -> (-18.7627, 38.8088) projected
  line L8 (-18.7627, 38.8088) -> (-19.1711, 40.1313) projected
  spline S4 degree 2 poles (-23.0745, 35.3784) (-23.2171, 35.44) (-23.4764, 35.4594) (-23.7001, 35.4594) knots 0 0 0 0.5 1 1 1 projected
  line L9 (-23.7001, 35.4594) -> (-23.8427, 35.4594) projected
  line L10 (-23.8427, 35.4594) -> (-23.8427, 34.2601) projected
  line L11 (-23.8427, 34.2601) -> (-23.7714, 34.2601) projected
  spline S5 degree 2 poles (-23.7714, 34.2601) (-23.632, 34.2601) (-23.3792, 34.2666) (-23.2852, 34.2828) knots 0 0 0 0.5 1 1 1 projected
  spline S6 degree 2 poles (-23.2852, 34.2828) (-23.2041, 34.2957) (-23.0258, 34.3735) (-22.9772, 34.4222) knots 0 0 0 0.5 1 1 1 projected
  spline S7 degree 2 poles (-22.9772, 34.4222) (-22.8735, 34.5194) (-22.8022, 34.7366) (-22.8022, 34.9181) knots 0 0 0 0.5 1 1 1 projected
  spline S8 degree 2 poles (-22.8022, 34.9181) (-22.8022, 35.0899) (-22.9642, 35.333) (-23.0745, 35.3784) knots 0 0 0 0.5 1 1 1 projected
  spline S9 degree 2 poles (-28.3646, 35.226) (-28.491, 35.3914) (-28.8151, 35.534) (-28.9902, 35.534) knots 0 0 0 0.5 1 1 1 projected
  spline S10 degree 2 poles (-28.9902, 35.534) (-29.1749, 35.534) (-29.4764, 35.4011) (-29.6158, 35.2325) knots 0 0 0 0.5 1 1 1 projected
  spline S11 degree 2 poles (-29.6158, 35.2325) (-29.739, 35.0769) (-29.8913, 34.5615) (-29.8913, 34.205) knots 0 0 0 0.5 1 1 1 projected
  spline S12 degree 2 poles (-29.8913, 34.205) (-29.8913, 33.8354) (-29.7454, 33.3492) (-29.619, 33.1839) knots 0 0 0 0.5 1 1 1 projected
  spline S13 degree 2 poles (-29.619, 33.1839) (-29.4926, 33.0186) (-29.1652, 32.876) (-28.9902, 32.876) knots 0 0 0 0.5 1 1 1 projected
  spline S14 degree 2 poles (-28.9902, 32.876) (-28.8119, 32.876) (-28.4813, 33.0283) (-28.3613, 33.1904) knots 0 0 0 0.5 1 1 1 projected
  spline S15 degree 2 poles (-28.3613, 33.1904) (-28.2317, 33.3654) (-28.0923, 33.829) (-28.0923, 34.205) knots 0 0 0 0.5 1 1 1 projected
  spline S16 degree 2 poles (-28.0923, 34.205) (-28.0923, 34.5648) (-28.2382, 35.0672) (-28.3646, 35.226) knots 0 0 0 0.5 1 1 1 projected
  spline S17 degree 2 poles (-29.4117, 29.5788) (-29.6159, 29.689) (-30.0633, 29.7117) (-30.3744, 29.7117) knots 0 0 0 0.5 1 1 1 projected
  line L12 (-30.3744, 29.7117) -> (-30.3939, 29.7117) projected
  line L13 (-30.3939, 29.7117) -> (-30.3939, 27.206) projected
  line L14 (-30.3939, 27.206) -> (-30.3744, 27.206) projected
  spline S18 degree 2 poles (-30.3744, 27.206) (-30.0373, 27.206) (-29.5738, 27.2287) (-29.3631, 27.3616) knots 0 0 0 0.5 1 1 1 projected
  spline S19 degree 2 poles (-29.3631, 27.3616) (-29.1168, 27.5172) (-28.8607, 28.065) (-28.8607, 28.4604) knots 0 0 0 0.5 1 1 1 projected
  spline S20 degree 2 poles (-28.8607, 28.4604) (-28.8607, 28.8559) (-29.133, 29.4199) (-29.4117, 29.5788) knots 0 0 0 0.5 1 1 1 projected
  spline S21 degree 2 poles (-17.6419, 28.4604) (-17.6419, 28.817) (-17.7877, 29.3194) (-17.9142, 29.4815) knots 0 0 0 0.5 1 1 1 projected
  spline S22 degree 2 poles (-17.9142, 29.4815) (-18.0406, 29.6436) (-18.3647, 29.7862) (-18.5398, 29.7862) knots 0 0 0 0.5 1 1 1 projected
  spline S23 degree 2 poles (-18.5398, 29.7862) (-18.7245, 29.7862) (-19.026, 29.6533) (-19.1654, 29.4848) knots 0 0 0 0.5 1 1 1 projected
  spline S24 degree 2 poles (-19.1654, 29.4848) (-19.2885, 29.3292) (-19.4409, 28.8138) (-19.4409, 28.4572) knots 0 0 0 0.5 1 1 1 projected
  spline S25 degree 2 poles (-19.4409, 28.4572) (-19.4409, 28.0909) (-19.295, 27.6047) (-19.1686, 27.4394) knots 0 0 0 0.5 1 1 1 projected
  spline S26 degree 2 poles (-19.1686, 27.4394) (-19.0422, 27.2741) (-18.7148, 27.1314) (-18.5398, 27.1314) knots 0 0 0 0.5 1 1 1 projected
  spline S27 degree 2 poles (-18.5398, 27.1314) (-18.3615, 27.1314) (-18.0309, 27.2838) (-17.9109, 27.4459) knots 0 0 0 0.5 1 1 1 projected
  spline S28 degree 2 poles (-17.9109, 27.4459) (-17.7813, 27.6209) (-17.6419, 28.0844) (-17.6419, 28.4604) knots 0 0 0 0.5 1 1 1 projected
  line L15 (-24.167, 29.3227) -> (-24.5787, 28.0002) projected
  line L16 (-24.5787, 28.0002) -> (-23.7586, 28.0002) projected
  line L17 (-23.7586, 28.0002) -> (-24.167, 29.3227) projected
  point P0 (0, 0)
  constraints: 29 other
extrude "Extrusion9" cut sketch "Sketch9" against normal blind 10
chamfer "Chamfer2" distance 1.8 angle 45 3 edges at (11.0671, 28.841, 2) (11.0671, 34.601, 2) (11.0671, 39.721, 2)
body "Solid1"
